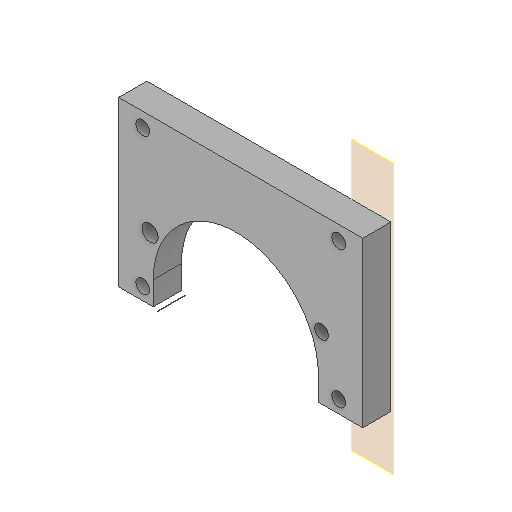
# Autodesk Inventor part: 20_Cube_Insert_Beamsplittercube_motorized_motormount
Saved by Autodesk Inventor 2022 (Build 260153000, 153)
## iProperties
Created: 2021-10-11
Part Number: 20_Cube_Insert_Beamsplittercube_motorized_motormount
Material: Generic
Document SubType Name: Modeling
Designer: diederichbenedict
Density: 1 g/cm^3
Appearance: Default
Author: diederichbenedict
Autodesk Inventor part; units mm, degrees
ref_plane "YZ Plane" through (0, 0, 0) normal (1, 0, 0) x (0, 1, 0)
ref_plane "Work Plane1" through (0, 0, 0) normal (0, 0, 1) x (1, 0, 0)
sketch "Sketch1" plane through (0, 0, 0) normal (0, 0, 1) x (1, 0, 0)
  circle A0 centre (-20, 14) radius 1.4 projected
  circle A1 centre (-20, -14) radius 1.4 projected
  circle A2 centre (20, -14) radius 1.4 projected
  circle A3 centre (20, 14) radius 1.4 projected
  line L0 (-24.9, 22.9) -> (-24.9, -22.9) projected
  line L1 (24.9, -22.9) -> (24.9, 22.9) projected
  line L2 (-24.9, 16.9002) -> (24.9, 16.9002)
  line L3 (24.9, 16.9002) -> (24.9, -16.5998)
  line L4 (-24.9, -16.5998) -> (-24.9, 16.9002)
  line L5 (-17.05, -17.05) -> (-17.05, 17.05) construction
  line L6 (17.05, 17.05) -> (17.05, -17.05) construction
  line L7 (-17.05, -17.05) -> (17.05, -17.05)
  line L8 (17.05, -17.05) -> (17.05, 4.95)
  line L9 (-17.05, 4.95) -> (-17.05, -17.05)
  circle A4 centre (-1, -11.8188) radius 15.5 construction
  line L10 (15.8586, -11.8188) -> (15.8586, -16.5998)
  line L11 (-17.8586, -11.8188) -> (-17.8586, -16.5998)
  arc A5 (15.8586, -11.8188) -> (-17.8586, -11.8188) centre (-1, -11.8188) ccw
  arc A6 (-17.05, -16.9773) -> (-17.0265, -17.05) centre (-1, -11.8188) ccw
  line L12 (24.9, -16.5998) -> (15.8586, -16.5998)
  line L13 (-17.8586, -16.5998) -> (-24.9, -16.5998)
  arc A7 (14.4, -3.8188) -> (18.6, -3.8188) centre (16.5, -3.8188) ccw construction
  arc A8 (-20.6, -3.8188) -> (-16.4, -3.8188) centre (-18.5, -3.8188) ccw construction
  circle A9 centre (-18.5, -3.8188) radius 1.6708
  circle A10 centre (16.5, -3.8188) radius 1.4
  dimension "d0" = 33.5
  dimension "d1" = 22
  dimension "d4" = 2.8
  dimension "d5" = 0
  constraints: 20 end point, 8 point on circle, 7 centre point, 6 perpendicular, 5 point on line, 4 parallel, 2 coincident, 2 horizontal, 2 tangent, 10 other
  measures "d0" distance of L2.end L3.end
  measures "d1" distance of L8.end L7.end
  measures "d4" diameter of A10
  measures "d5" distance between parallel lines of L13 L12
ref_plane "Work Plane2" through (-22, -17.8188, 7.2556) normal (0, 0, 1) x (1, 0, 0)
ref_plane "Work Plane3" through (-22, -17.8188, 5.7556) normal (0, 0, 1) x (1, 0, 0)
extrude "Extrusion1" add sketch "Sketch1" along normal up to surface (5.7556 mm away) contours L2 L1 L12 L10 A5 L11 L13 L0 | A6 L7 L9
body "Solid1"
